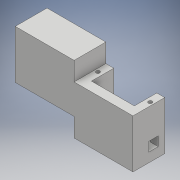
# Autodesk Inventor part: FEMUR
Saved by Autodesk Inventor 2017 (Build 210142000, 142)
## iProperties
Created: 2018-01-06
Part Number: FEMUR
Material: Generic
Document SubType Name: Modeling
Designer: Alex
Density: 1 g/cm^3
Appearance: Default
Author: Alex
Autodesk Inventor part; units mm, degrees
ref_plane "YZ Plane" through (0, 0, 0) normal (1, 0, 0) x (0, 1, 0)
ref_plane "XZ Plane" through (0, 0, 0) normal (0, 1, 0) x (-1, 0, 0)
ref_plane "XY Plane" through (0, 0, 0) normal (0, 0, 1) x (1, 0, 0)
sketch "Sketch1" plane through (0, 0, 0) normal (0, 1, 0) x (-1, 0, 0)
  line L0 (31.5, 18) -> (0, 18)
  line L1 (0, 18) -> (0, -8)
  line L2 (0, -8) -> (31.5, -8)
  line L3 (31.5, -8) -> (31.5, 18)
  line L4 (0, -25.2) -> (0, 25.2) projected
  line L5 (-31.5, -18) -> (0, -18)
  line L6 (0, -18) -> (0, 8)
  line L7 (0, 8) -> (-31.5, 8)
  line L8 (-31.5, 8) -> (-31.5, -18)
  point P0 (0, 0)
  dimension "d1" = 31.5
  dimension "d7" = 360
  dimension "d9" = 26
  dimension "d11" = 16
  constraints: 16 end point, 2 parallel, 1 collinear, 1 horizontal, 1 perpendicular, 17 other
  measures "d1" distance of L1.end L2.end
  measures "d9" distance of L2.end L0.start
  measures "d11" distance between parallel lines of L7 L2
extrude "Extrusion1" add sketch "Sketch1" along normal blind 17
sketch "Sketch3" plane through (0, 17, 0) normal (0, 1, 0) x (1, 0, 0)
  line L0 (-27.25, 8) -> (-4.25, 8)
  line L1 (-4.25, 8) -> (-4.25, -13)
  line L2 (-4.25, -13) -> (-27.25, -13)
  line L3 (-27.25, -13) -> (-27.25, 8)
  line L4 (27.25, -8) -> (4.25, -8)
  line L5 (4.25, -8) -> (4.25, 13)
  line L6 (4.25, 13) -> (27.25, 13)
  line L7 (27.25, 13) -> (27.25, -8)
  line L8 (0, 8) -> (-31.5, 8) projected
  line L9 (-31.5, -18) -> (0, -18) projected
  line L10 (-31.5, 8) -> (-31.5, -18) projected
  line L11 (0, -18) -> (0, -8) projected
  point P0 (0, 0)
  dimension "d16" = 360
  dimension "d19" = 4.25
  dimension "d20" = 4.25
  dimension "d33" = 5
  constraints: 16 end point, 2 parallel, 1 collinear, 1 horizontal, 1 perpendicular, 17 other
  measures "d19" distance between parallel lines of L10 L3
  measures "d20" distance between parallel lines of L11 L1
  measures "d33" distance between parallel lines of L9 L2
extrude "Extrusion2" cut sketch "Sketch3" against normal blind 12
sketch "Sketch6" plane through (0, 0, -8) normal (0, 0, -1) x (-1, 0, 0)
  circle A0 centre (29.75, 11) radius 1
  circle A1 centre (1.75, 11) radius 1
  line L0 (4.25, 5) -> (4.25, 17) projected
  line L1 (27.25, 17) -> (27.25, 5) projected
  point P0 (0, 0)
  point P1 (4.25, 11)
  dimension "d35" = 1.5
  dimension "d36" = 2
  dimension "d37" = 1.5
  constraints: 2 centre point, 2 horizontal alignment, 1 equal radius, 1 midpoint
  measures "d35" distance edge to line of A1 L0
  measures "d36" diameter of A1
  measures "d37" distance edge to line of A0 L1
extrude "Extrusion5" cut sketch "Sketch6" against normal blind 10
sketch "Sketch7" plane through (0, 0, 8) normal (0, 0, 1) x (1, 0, 0)
  circle A0 centre (1.75, 11) radius 1
  circle A1 centre (29.75, 11) radius 1
  line L0 (27.25, 17) -> (27.25, 5) projected
  line L1 (4.25, 5) -> (4.25, 17) projected
  point P0 (0, 0)
  point P1 (27.25, 11)
  dimension "d40" = 2
  dimension "d41" = 1.5
  dimension "d42" = 1.5
  constraints: 2 centre point, 2 horizontal alignment, 1 equal radius, 1 midpoint
  measures "d40" diameter of A1
  measures "d41" distance edge to line of A1 L0
  measures "d42" distance edge to line of A0 L1
extrude "Extrusion6" cut sketch "Sketch7" against normal blind 10
sketch "Sketch8" plane through (31.5, 0, 8) normal (1, 0, 0) x (0, 0, -1)
  line L0 (21, 17) -> (21, 5) projected
  line L1 (21, 5) -> (0, 5) projected
  line L2 (21, 13.5) -> (16, 13.5)
  line L3 (16, 13.5) -> (16, 8.5)
  line L4 (16, 8.5) -> (21, 8.5)
  line L5 (21, 8.5) -> (21, 13.5)
  point P0 (8, 0)
  point P1 (21, 11)
  point P2 (21, 11)
  dimension "d45" = 5
  dimension "d47" = 5
  constraints: 8 end point, 2 midpoint, 2 parallel, 1 coincident, 1 collinear, 1 horizontal, 1 perpendicular
  measures "d45" distance of L2.end L3.end
  measures "d47" distance of L3.end L4.end
extrude "Extrusion7" cut sketch "Sketch8" against normal up to surface (4.25 mm away)
sketch "Sketch9" plane through (-31.5, 0, -8) normal (-1, 0, 0) x (0, 0, 1)
  line L0 (21, 17) -> (21, 5) projected
  line L1 (21, 5) -> (0, 5) projected
  line L2 (21, 8.5) -> (16, 8.5)
  line L3 (16, 8.5) -> (16, 13.5)
  line L4 (16, 13.5) -> (21, 13.5)
  line L5 (21, 13.5) -> (21, 8.5)
  point P0 (8, 0)
  point P1 (21, 11)
  point P2 (21, 11)
  dimension "d50" = 5
  dimension "d51" = 5
  constraints: 8 end point, 2 midpoint, 2 parallel, 1 coincident, 1 collinear, 1 horizontal, 1 perpendicular
  measures "d50" distance of L2.end L3.end
  measures "d51" distance of L3.end L4.end
extrude "Extrusion8" cut sketch "Sketch9" against normal up to surface (4.25 mm away)
equation "\"d1\" = servo_D"
equation "\"d9\" = servo_E + mat"
equation "\"d12\" = servo_B + mat"
equation "\"d19\" = -0.5 * servo_A + 0.5 * servo_D"
equation "\"d20\" = d19"
equation "\"d33\" = mat"
equation "\"d21\" = servo_B"
equation "\"d35\" = servo_L"
equation "\"d36\" = servo_H"
equation "\"d37\" = servo_L"
equation "\"d40\" = servo_H"
equation "\"d41\" = servo_L"
equation "\"d42\" = servo_L"
equation "\"d45\" = servo_K"
equation "\"d47\" = servo_K"
equation "\"d50\" = servo_K"
equation "\"d51\" = servo_K"
equation "\"mat\" = 5"
equation "\"servo_D\" = 31.5"
equation "\"servo_E\" = 21"
equation "\"servo_B\" = 12"
equation "\"servo_A\" = 23"
equation "\"servo_L\" = 1.5"
equation "\"servo_H\" = 2"
equation "\"servo_K\" = 5"
body "Solid1"
